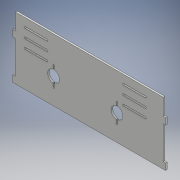
# Autodesk Inventor part: flipper-support
Saved by Autodesk Inventor 2017 (Build 210142000, 142)
## iProperties
Created: 2017-03-05
Part Number: flipper-support
Material: Generic
Document SubType Name: Modeling
Designer: John
Density: 1 g/cm^3
Appearance: Default
Author: John
Autodesk Inventor part; units mm, degrees
ref_plane "YZ Plane" through (0, 0, 0) normal (1, 0, 0) x (0, 1, 0)
ref_plane "XZ Plane" through (0, 0, 0) normal (0, 1, 0) x (-1, 0, 0)
ref_plane "XY Plane" through (0, 0, 0) normal (0, 0, 1) x (1, 0, 0)
sketch "Sketch1" plane through (0, 0, 0) normal (0, 1, 0) x (-1, 0, 0)
  line L0 (0, 0) -> (271, 0)
  line L1 (271, 0) -> (271, 84)
  line L2 (271, 84) -> (0, 84)
  line L3 (0, 84) -> (0, 0)
  line L4 (135.5, 84) -> (135.5, 0) construction
  line L5 (0, 84) -> (-4, 84)
  line L6 (-4, 84) -> (-4, 72)
  line L7 (-4, 72) -> (0, 72)
  line L8 (0, 72) -> (0, 84)
  line L9 (0, 0) -> (-4, 0)
  line L10 (-4, 0) -> (-4, 12)
  line L11 (-4, 12) -> (0, 12)
  line L12 (0, 12) -> (0, 0)
  line L13 (271, 84) -> (271, 0)
  line L14 (271, 84) -> (275, 84)
  line L15 (275, 84) -> (275, 72)
  line L16 (275, 72) -> (271, 72)
  line L17 (271, 72) -> (271, 84)
  line L18 (271, 0) -> (275, 0)
  line L19 (275, 0) -> (275, 12)
  line L20 (275, 12) -> (271, 12)
  line L21 (271, 12) -> (271, 0)
  line L22 (200.5, 46.871) -> (84.5, 46.871) construction
  circle A0 centre (200.5, 46.871) radius 10.825
  arc A1 (201.5, 64.696) -> (199.5, 64.696) centre (200.5, 64.696) ccw
  line L23 (200.5, 57.696) -> (200.5, 64.696) construction
  line L24 (201.5, 57.696) -> (201.5, 64.696)
  line L25 (199.5, 64.696) -> (199.5, 57.696)
  arc A2 (199.5, 57.696) -> (201.5, 57.696) centre (200.5, 57.696) ccw
  arc A3 (201.5, 36.046) -> (199.5, 36.046) centre (200.5, 36.046) ccw
  line L26 (201.5, 29.046) -> (201.5, 36.046)
  arc A4 (199.5, 29.046) -> (201.5, 29.046) centre (200.5, 29.046) ccw
  line L27 (200.5, 36.046) -> (200.5, 29.046) construction
  line L28 (199.5, 36.046) -> (199.5, 29.046)
  arc A5 (85.5, 36.046) -> (83.5, 36.046) centre (84.5, 36.046) ccw
  arc A6 (83.5, 57.696) -> (85.5, 57.696) centre (84.5, 57.696) ccw
  line L29 (83.5, 64.696) -> (83.5, 57.696)
  line L30 (84.5, 57.696) -> (84.5, 64.696) construction
  line L31 (85.5, 57.696) -> (85.5, 64.696)
  arc A7 (85.5, 64.696) -> (83.5, 64.696) centre (84.5, 64.696) ccw
  circle A8 centre (84.5, 46.871) radius 10.825
  arc A9 (83.5, 29.046) -> (85.5, 29.046) centre (84.5, 29.046) ccw
  line L32 (83.5, 36.046) -> (83.5, 29.046)
  line L33 (84.5, 36.046) -> (84.5, 29.046) construction
  line L34 (85.5, 29.046) -> (85.5, 36.046)
  point P0 (200.5, 61.196)
  point P1 (200.5, 32.546)
  point P2 (84.5, 46.871)
  point P3 (84.5, 61.196)
  point P4 (84.5, 32.546)
  dimension "d0" = 271
  dimension "d1" = 84
  dimension "d2" = 4
  dimension "d3" = 12
  dimension "d4" = 4
  dimension "d5" = 12
  dimension "d11" = 116
  dimension "d13" = 37.129
  dimension "d14" = 84.5
  dimension "d15" = 21.65
  dimension "d16" = 7
  dimension "d17" = 2
  dimension "d18" = 7
  dimension "d19" = 2
  dimension "d20" = 21.65
  dimension "d21" = 7
  dimension "d22" = 2
  dimension "d23" = 7
  dimension "d24" = 2
  constraints: 78 end point, 20 point on circle, 16 tangent, 10 centre point, 10 parallel, 6 midpoint, 6 symmetric about line, 4 horizontal, 4 vertical, 3 perpendicular, 2 coincident
  measures "d0" distance of L2.end L1.end
  measures "d1" distance of L1.end L0.end
  measures "d2" distance of L7.end L6.end
  measures "d3" distance of L6.end L5.end
  measures "d4" distance of L10.end L11.end
  measures "d5" distance of L9.end L10.end
  measures "d11" distance of L22.end L22.start
  measures "d13" distance from line of L2 L22.start
  measures "d14" distance from line of L3 L22.end
  measures "d15" diameter of A0
  measures "d16" distance of L23.start L23.end
  measures "d17" diameter of A1
  measures "d18" distance of L27.start L27.end
  measures "d19" diameter of A4
  measures "d20" diameter of A8
  measures "d21" distance of L30.start L30.end
  measures "d22" diameter of A7
  measures "d23" distance of L33.start L33.end
  measures "d24" diameter of A9
extrude "Extrusion1" add sketch "Sketch1" along normal blind 3
sketch "Sketch3" plane through (0, 0, 0) normal (0, -1, 0) x (1, 0, 0)
  line L0 (4, 0) -> (-275, 0) projected
  line L1 (-270, 114) -> (0, 114)
  line L2 (0, 114) -> (0, 84)
  line L3 (0, 84) -> (-270, 84)
  line L4 (-270, 84) -> (-270, 114)
  line L5 (-275, 84) -> (4, 84) projected
  point P0 (0, 0)
  dimension "d28" = 30
  constraints: 8 end point, 2 parallel, 1 collinear, 1 horizontal, 1 perpendicular
  measures "d28" distance of L1.end L2.end
extrude "Extrusion2" add sketch "Sketch3" against normal blind 3
sketch "Sketch2" plane through (0, 0, 0) normal (0, -1, 0) x (1, 0, 0)
  circle A0 centre (-232.5, 81.871) radius 1.5 construction
  arc A1 (-199.5011, 36.0922) -> (-199.5011, 57.6498) centre (-200.5, 46.871) ccw projected
  circle A2 centre (-251.5, 81.871) radius 1.5 construction
  circle A3 centre (-251.5, 98.371) radius 1.5 construction
  circle A4 centre (-232.5, 98.371) radius 1.5 construction
  line L0 (-251.5, 98.371) -> (-232.5, 98.371) construction
  line L1 (-251.5, 98.371) -> (-251.5, 81.871) construction
  line L2 (-252.5, 98.371) -> (-212.5, 98.371) construction
  line L3 (-252.5, 96.871) -> (-212.5, 96.871)
  line L4 (-212.5, 99.871) -> (-252.5, 99.871)
  arc A5 (-252.5, 99.871) -> (-252.5, 96.871) centre (-252.5, 98.371) ccw
  arc A6 (-212.5, 96.871) -> (-212.5, 99.871) centre (-212.5, 98.371) ccw
  line L5 (-252.5, 81.871) -> (-212.5, 81.871) construction
  line L6 (-252.5, 80.371) -> (-212.5, 80.371)
  line L7 (-212.5, 83.371) -> (-252.5, 83.371)
  arc A7 (-252.5, 83.371) -> (-252.5, 80.371) centre (-252.5, 81.871) ccw
  arc A8 (-212.5, 80.371) -> (-212.5, 83.371) centre (-212.5, 81.871) ccw
  circle A9 centre (-52.5, 81.871) radius 1.5 construction
  arc A10 (-83.5011, 36.0922) -> (-83.5011, 57.6498) centre (-84.5, 46.871) ccw construction
  line L8 (-32.5, 81.871) -> (-72.5, 81.871) construction
  line L9 (-32.5, 83.371) -> (-72.5, 83.371)
  line L10 (-72.5, 80.371) -> (-32.5, 80.371)
  arc A11 (-32.5, 80.371) -> (-32.5, 83.371) centre (-32.5, 81.871) ccw
  arc A12 (-72.5, 83.371) -> (-72.5, 80.371) centre (-72.5, 81.871) ccw
  line L11 (-32.5, 98.371) -> (-72.5, 98.371) construction
  line L12 (-32.5, 99.871) -> (-72.5, 99.871)
  line L13 (-72.5, 96.871) -> (-32.5, 96.871)
  arc A13 (-32.5, 96.871) -> (-32.5, 99.871) centre (-32.5, 98.371) ccw
  arc A14 (-72.5, 99.871) -> (-72.5, 96.871) centre (-72.5, 98.371) ccw
  line L14 (-252.5, 65.371) -> (-212.5, 65.371) construction
  line L15 (-252.5, 63.871) -> (-212.5, 63.871)
  line L16 (-212.5, 66.871) -> (-252.5, 66.871)
  arc A15 (-252.5, 66.871) -> (-252.5, 63.871) centre (-252.5, 65.371) ccw
  arc A16 (-212.5, 63.871) -> (-212.5, 66.871) centre (-212.5, 65.371) ccw
  line L17 (-212.5, 81.871) -> (-212.5, 65.371) construction
  line L18 (-32.5, 65.371) -> (-72.5, 65.371) construction
  line L19 (-32.5, 66.871) -> (-72.5, 66.871)
  line L20 (-72.5, 63.871) -> (-32.5, 63.871)
  arc A17 (-32.5, 63.871) -> (-32.5, 66.871) centre (-32.5, 65.371) ccw
  arc A18 (-72.5, 66.871) -> (-72.5, 63.871) centre (-72.5, 65.371) ccw
  line L21 (-72.5, 81.871) -> (-72.5, 65.371) construction
  line L22 (-72.5, 98.371) -> (-72.5, 81.871) construction
  point P0 (0, 0)
  point P1 (-52.5, 98.371)
  point P2 (-232.5, 65.371)
  point P3 (-52.5, 65.371)
  dimension "d25" = 3
  dimension "d26" = 32
  dimension "d27" = 35
  dimension "d31" = 3
  dimension "d32" = 3
  dimension "d33" = 3
  dimension "d34" = 19
  dimension "d35" = 16.5
  dimension "d38" = 20
  dimension "d39" = 20
  dimension "d40" = 3
  dimension "d41" = 3
  dimension "d43" = 32
  dimension "d44" = 35
  dimension "d45" = 20
  dimension "d46" = 3
  dimension "d47" = 20
  dimension "d48" = 3
  dimension "d49" = 20
  dimension "d50" = 3
  dimension "d51" = 16.5
  dimension "d52" = 20
  dimension "d53" = 3
  dimension "d54" = 16.5
  constraints: 58 end point, 24 point on circle, 24 tangent, 17 centre point, 7 parallel, 6 horizontal, 6 midpoint, 3 vertical, 1 collinear, 1 perpendicular
  measures "d25" diameter of A0
  measures "d26" horizontal distance of A1.centre A0.centre
  measures "d27" vertical distance of A0.centre A1.centre
  measures "d31" diameter of A2
  measures "d32" diameter of A3
  measures "d33" diameter of A4
  measures "d34" distance of A0.centre L1.end
  measures "d35" distance of A0.centre L0.end
  measures "d38" distance of L0.end L2.end
  measures "d39" distance of A0.centre L5.end
  measures "d40" diameter of A8
  measures "d41" diameter of A9
  measures "d43" horizontal distance of A10.centre A9.centre
  measures "d44" vertical distance of A10.centre A9.centre
  measures "d45" distance of A9.centre L8.end
  measures "d46" diameter of A12
  measures "d47" distance of point (-52.5, 98.371) L11.end
  measures "d48" diameter of A14
  measures "d49" distance of point (-232.5, 65.371) L14.end
  measures "d50" diameter of A16
  measures "d51" distance of L5.end L14.end
  measures "d52" distance of point (-52.5, 65.371) L18.end
  measures "d53" diameter of A18
  measures "d54" distance between parallel lines of L8 L18
extrude "Extrusion3" cut sketch "Sketch2" against normal blind 3
equation "\"d4\" = d2"
equation "\"d31\" = d25"
equation "\"d32\" = d25"
equation "\"d33\" = d25"
equation "\"d41\" = d40"
equation "\"d43\" = d26"
equation "\"d44\" = d27"
body "Solid1"
